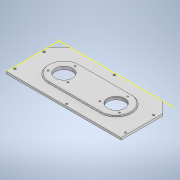
# Autodesk Inventor part: tampa da carcaça terminada 1
Saved by Autodesk Inventor 2022.1 (Build 261234020, 234B)
## iProperties
Created: 2023-09-12
Part Number: tampa da carcaça terminada 1
Material: Generic
Document SubType Name: Modeling
Designer: SENAI
Density: 1 g/cm^3
Appearance: Default
Author: SENAI
Autodesk Inventor part; units mm, degrees
ref_plane "YZ Plane" through (0, 0, 0) normal (1, 0, 0) x (0, 1, 0)
ref_plane "XZ Plane" through (0, 0, 0) normal (0, 1, 0) x (-1, 0, 0)
ref_plane "XY Plane" through (0, 0, 0) normal (0, 0, 1) x (1, 0, 0)
sketch "Sketch1" plane through (0, 0, 0) normal (0, 0, 1) x (1, 0, 0)
  line L0 (0, 0) -> (460, 0)
  line L1 (460, 0) -> (460, 9)
  line L2 (460, 9) -> (0, 9)
  line L3 (0, 9) -> (0, 0)
  dimension "d0" = 460
  dimension "d1" = 9
  constraints: 8 end point, 2 parallel, 1 horizontal, 1 perpendicular
  measures "d0" distance of L2.end L1.end
  measures "d1" distance of L1.end L0.end
extrude "Extrusion1" add sketch "Sketch1" along normal blind 211
sketch "Sketch2" plane through (0, 9, 0) normal (0, 1, 0) x (1, 0, 0)
  line L0 (460, 0) -> (0, 0) projected
  line L1 (460, -211) -> (0, -211) projected
  line L2 (0, 0) -> (0, -211) projected
  circle A0 centre (125.25, -105.5) radius 34.75
  circle A1 centre (334.75, -105.5) radius 34.75
  arc A2 (125.25, -43.25) -> (125.25, -167.75) centre (125.25, -105.5) ccw
  arc A3 (334.75, -167.75) -> (334.75, -43.25) centre (334.75, -105.5) ccw
  line L3 (125.25, -43.25) -> (334.75, -43.25)
  line L4 (125.25, -167.75) -> (334.75, -167.75)
  point P0 (230, -105.5)
  dimension "d6" = 69.5
  dimension "d7" = 69.5
  constraints: 4 centre point, 4 end point, 4 point on circle, 2 coincident, 1 horizontal, 1 tangent
  measures "d6" diameter of A0
  measures "d7" diameter of A1
extrude "Extrusion2" add sketch "Sketch2" along normal blind 3.5
sketch "Sketch3" plane through (125.25, 9, 105.5) normal (0, 1, 0) x (1, 0, 0)
  circle A0 centre (0, 0) radius 34.75
  circle A1 centre (209.2921, 0) radius 34.75
  point P0 (-125.25, 105.5)
  dimension "d12" = 69.5
  dimension "d13" = 69.5
  constraints: 2 centre point
  measures "d12" diameter of A0
  measures "d13" diameter of A1
extrude "Extrusion3" cut sketch "Sketch3" against normal through all
fillet "Fillet1" radius 3 4 edges at (397, 12.5, 105.5) (230, 12.5, 43.25) (63, 12.5, 105.5) (230, 12.5, 167.75) inverted yes
sketch "Sketch4" plane through (0, 9, 0) normal (0, 1, 0) x (1, 0, 0)
  circle A0 centre (230, -8) radius 4
  line L0 (460, 0) -> (0, 0) projected
  circle A1 centre (234.1267, -202.9944) radius 4
  circle A2 centre (8.4984, -68.1147) radius 4
  circle A3 centre (447.5, -68.1147) radius 4
  circle A4 centre (451.5, -184.9999) radius 4
  circle A5 centre (8.4984, -185.1147) radius 4
  line L1 (460, -211) -> (0, -211) projected
  line L2 (0, 0) -> (0, -211) projected
  line L3 (460, 0) -> (460, -211) projected
  line L4 (0, -39.1147) -> (55.3165, -39.1147) construction
  point P0 (230, -105.5)
  dimension "d17" = 8
  dimension "d20" = 8
  dimension "d22" = 8
  dimension "d23" = 8
  dimension "d24" = 8
  dimension "d25" = 8
  constraints: 6 centre point, 2 end point, 1 horizontal, 1 point on line
  measures "d17" diameter of A0
  measures "d20" diameter of A1
  measures "d22" diameter of A2
  measures "d23" diameter of A3
  measures "d24" diameter of A4
  measures "d25" diameter of A5
extrude "Extrusion4" cut sketch "Sketch4" against normal through all contours A0 | A1 | A2 | A3 | A4 | A5
sketch "Sketch5" plane through (0, 9, 0) normal (0, 1, 0) x (1, 0, 0)
  line L0 (0, 0) -> (0, -211) projected
  line L1 (0, 0) -> (460, 0) projected
chamfer "Chamfer1" distance 43.5 angle 45 2 edges at (0, 4.5, 0) (460, 4.5, 0)
sketch "Sketch6" plane through (0, 12.5, 0) normal (0, 1, 0) x (1, 0, 0)
  point P0 (0, 0)
sketch "Sketch7" plane through (0, 12.5, 0) normal (0, 1, 0) x (1, 0, 0)
  point P0 (0, 0)
sketch "Sketch8" plane through (0, 12.5, 0) normal (0, 1, 0) x (1, 0, 0)
  circle A0 centre (123.8213, -58.75) radius 3
  circle A1 centre (165.2981, -129.6135) radius 3
  circle A2 centre (84.4784, -128.372) radius 3
  circle A3 centre (334.6461, -58.7502) radius 3
  circle A4 centre (295.4929, -131.1557) radius 3
  circle A5 centre (373.7401, -131.2415) radius 3
  arc A6 (334.6461, -70.7502) -> (334.6461, -140.2498) centre (334.5421, -105.5) ccw projected
  circle A7 centre (334.75, -105.5) radius 34.75 projected
  circle A8 centre (125.25, -105.5) radius 34.75 projected
  point P0 (0, 0)
  dimension "d43" = 6
  dimension "d44" = 6
  dimension "d45" = 6
  dimension "d46" = 6
  dimension "d47" = 6
  dimension "d48" = 6
  constraints: 6 centre point
  measures "d43" diameter of A0
  measures "d44" diameter of A1
  measures "d45" diameter of A2
  measures "d46" diameter of A3
  measures "d47" diameter of A4
  measures "d48" diameter of A5
extrude "Extrusion5" cut sketch "Sketch8" against normal through all contours A0 | A1 | A2 | A3 | A4 | A5
sketch "Sketch9" plane through (0, 9, 211) normal (0, 1, 0) x (1, 0, 0)
  point P0 (0, 211)
body "Solid1"
